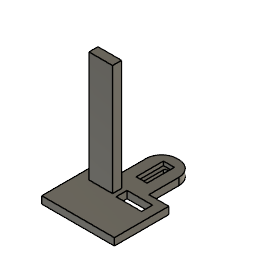
gripperForLego (Autodesk Fusion 360 design; units mm, degrees)
part number: 2026-06-01-16-59-25-849
Autodesk Fusion 360 part; units mm, degrees
sketch "スケッチ1" plane through (0, 0, 0) normal (0, 0, 1) x (1, 0, 0)
  line L0 (0, 0) -> (40, 0)
  line L1 (40, 0) -> (40, 30)
  line L2 (40, 30) -> (0, 30)
  line L3 (0, 30) -> (0, 0)
  line L4 (6, 21) -> (18, 21)
  line L5 (18, 21) -> (18, 25)
  line L6 (18, 25) -> (6, 25)
  line L7 (6, 25) -> (6, 21)
  line L8 (21, 20) -> (35, 20)
  line L9 (35, 20) -> (35, 26)
  line L10 (35, 26) -> (21, 26)
  line L11 (21, 26) -> (21, 20)
  dimension "d1" = 30
  constraint horizontal L0
  constraint vertical L1
  constraint horizontal L2
  constraint vertical L3
  constraint coincident L0.start L3.end
  constraint horizontal L4
  constraint vertical L5
  constraint horizontal L6
  constraint vertical L7
  constraint horizontal L8
  constraint vertical L9
  constraint horizontal L10
  constraint vertical L11
  measures "d1" distance of L0.end L1.end
extrude "押し出し1" add sketch "スケッチ1" along normal blind 4
sketch "スケッチ2" plane through (0, 0, 4) normal (0, 0, 1) x (-1, 0, 0)
  line L0 (-6, -21) -> (-6, -25)
  line L1 (-6, -25) -> (-18, -25)
  line L2 (-18, -25) -> (-18, -21)
  line L3 (-18, -21) -> (-6, -21)
  line L4 (-21, -20) -> (-21, -26)
  line L5 (-21, -26) -> (-35, -26)
  line L6 (-35, -26) -> (-35, -20)
  line L7 (-35, -20) -> (-21, -20)
  line L8 (0, -30) -> (0, 0)
  line L9 (0, 0) -> (-40, 0)
  line L10 (-40, 0) -> (-40, -30)
  line L11 (-40, -30) -> (0, -30)
sketch "スケッチ3" plane through (0, 0, 0) normal (0, 0, -1) x (1, 0, 0)
  line L0 (6, -25) -> (6, -21)
  line L1 (6, -21) -> (18, -21)
  line L2 (18, -21) -> (18, -25)
  line L3 (18, -25) -> (6, -25)
  line L4 (21, -26) -> (21, -20)
  line L5 (21, -20) -> (35, -20)
  line L6 (35, -20) -> (35, -26)
  line L7 (35, -26) -> (21, -26)
  line L8 (0, 0) -> (0, -30)
  line L9 (0, -30) -> (40, -30)
  line L10 (40, -30) -> (40, 0)
  line L11 (40, 0) -> (0, 0)
  line L12 (19, -21) -> (5, -21)
  line L13 (5, -21) -> (5, -26)
  line L14 (5, -26) -> (19, -26)
  line L15 (19, -26) -> (19, -21)
  constraint horizontal L12
  constraint vertical L13
  constraint horizontal L14
  constraint vertical L15
extrude "押し出し2" cut sketch "スケッチ3" against normal blind 1 contours L0 L2 L3 L12 L13 L14 L15
sketch "スケッチ4" plane through (0, 0, 0) normal (0, 0, -1) x (1, 0, 0)
  line L0 (0, 0) -> (0, -30)
  line L1 (0, -30) -> (40, -30)
  line L2 (40, -30) -> (40, 0)
  line L3 (40, 0) -> (0, 0)
  line L4 (21, -26) -> (21, -20)
  line L5 (21, -20) -> (35, -20)
  line L6 (35, -20) -> (35, -26)
  line L7 (35, -26) -> (21, -26)
  line L8 (5, -21) -> (19, -21)
  line L9 (19, -21) -> (19, -26)
  line L10 (19, -26) -> (5, -26)
  line L11 (5, -26) -> (5, -21)
sketch "スケッチ5" plane through (0, 0, 0) normal (0, 0, -1) x (1, 0, 0)
  line L0 (11, -30) -> (29, -30)
  line L1 (29, -30) -> (29, -55)
  line L2 (29, -55) -> (11, -55)
  line L3 (11, -55) -> (11, -30)
  line L4 (19, -48) -> (19, -37)
  line L5 (21, -48) -> (21, -37)
  circle A0 centre (20, -48) radius 1
  circle A1 centre (20, -37) radius 1
  constraint horizontal L0
  constraint vertical L1
  constraint horizontal L2
  constraint vertical L3
  constraint parallel L3 L4
  constraint vertical L5
  constraint coincident L5.start A0
  constraint tangent L5 A0
  constraint coincident L5.end A1
  constraint tangent L5 A1
extrude "押し出し3" add sketch "スケッチ5" against normal blind 4
fillet "フィレット1" radius 8.5 2 edges at (11, 55, 2) (29, 55, 2)
sketch "スケッチ6" plane through (0, 0, 4) normal (0, 0, 1) x (-1, 0, 0)
  line L0 (-19, -21) -> (-5, -21)
  line L1 (-5, -21) -> (-5, -26)
  line L2 (-5, -26) -> (-19, -26)
  line L3 (-19, -26) -> (-19, -21)
  constraint horizontal L0
  constraint vertical L1
  constraint horizontal L2
  constraint vertical L3
extrude "押し出し4" cut sketch "スケッチ6" against normal blind 2
extrude "押し出し5" add sketch "スケッチ4" against normal blind 1 contours L8 L9 L10 L11
extrude "押し出し6" cut sketch "スケッチ2" against normal blind 200 contours L0 L1 L2 L3
sketch "スケッチ7" plane through (0, 0, 4) normal (0, 0, 1) x (-1, 0, 0)
  line L0 (-19, -21) -> (-5, -21)
  line L1 (-5, -21) -> (-5, -26)
  line L2 (-5, -26) -> (-19, -26)
  line L3 (-19, -26) -> (-19, -21)
  arc A0 (-29, -46.5) -> (-20.5, -55) centre (-20.5, -46.5) ccw
  line L4 (-20.5, -55) -> (-19.5, -55)
  arc A1 (-19.5, -55) -> (-11, -46.5) centre (-19.5, -46.5) ccw
  line L5 (-11, -46.5) -> (-11, -30)
  line L6 (-11, -30) -> (0, -30)
  line L7 (0, -30) -> (0, 0)
  line L8 (0, 0) -> (-40, 0)
  line L9 (-40, 0) -> (-40, -30)
  line L10 (-40, -30) -> (-29, -30)
  line L11 (-29, -30) -> (-29, -46.5)
  arc A2 (-21, -48) -> (-19, -48) centre (-20, -48) ccw
  line L12 (-21, -48) -> (-21, -37)
  arc A3 (-19, -37) -> (-21, -37) centre (-20, -37) ccw
  line L13 (-19, -37) -> (-19, -48)
  line L14 (-21, -20) -> (-21, -26)
  line L15 (-21, -26) -> (-35, -26)
  line L16 (-35, -26) -> (-35, -20)
  line L17 (-35, -20) -> (-21, -20)
  line L18 (-17, -50) -> (-23, -50)
  line L19 (-23, -50) -> (-23, -35)
  line L20 (-23, -35) -> (-17, -35)
  line L21 (-17, -35) -> (-17, -50)
  constraint horizontal L18
  constraint vertical L19
  constraint horizontal L20
  constraint vertical L21
extrude "押し出し7" cut sketch "スケッチ7" against normal blind 2.2 contours L18 L19 L20 L21
sketch "スケッチ8" plane through (0, 0, 0) normal (0, 0, -1) x (1, 0, 0)
  line L0 (18, -25) -> (6, -25)
  line L1 (6, -25) -> (6, -21)
  line L2 (6, -21) -> (18, -21)
  line L3 (18, -21) -> (18, -25)
  arc A0 (19, -48) -> (21, -48) centre (20, -48) ccw
  line L4 (19, -48) -> (19, -37)
  arc A1 (21, -37) -> (19, -37) centre (20, -37) ccw
  line L5 (21, -37) -> (21, -48)
  arc A2 (20.5, -55) -> (29, -46.5) centre (20.5, -46.5) ccw
  line L6 (29, -46.5) -> (29, -30)
  line L7 (29, -30) -> (40, -30)
  line L8 (40, -30) -> (40, 0)
  line L9 (40, 0) -> (0, 0)
  line L10 (0, 0) -> (0, -30)
  line L11 (0, -30) -> (11, -30)
  line L12 (11, -30) -> (11, -46.5)
  arc A3 (11, -46.5) -> (19.5, -55) centre (19.5, -46.5) ccw
  line L13 (19.5, -55) -> (20.5, -55)
  line L14 (21, -26) -> (21, -20)
  line L15 (21, -20) -> (35, -20)
  line L16 (35, -20) -> (35, -26)
  line L17 (35, -26) -> (21, -26)
  line L18 (18.5, -25.5) -> (5.5, -25.5)
  line L19 (5.5, -25.5) -> (5.5, -20.5)
  line L20 (5.5, -20.5) -> (18.5, -20.5)
  line L21 (18.5, -20.5) -> (18.5, -25.5)
  line L22 (5, -26) -> (19, -26)
  line L23 (19, -26) -> (19, -21)
  line L24 (19, -21) -> (5, -21)
  line L25 (5, -21) -> (5, -26)
  constraint horizontal L18
  constraint vertical L19
  constraint horizontal L20
  constraint vertical L21
  constraint horizontal L22
  constraint vertical L23
  constraint horizontal L24
  constraint vertical L25
extrude "押し出し8" add 1 faces at (10, 25.6667, 2) along direction (0, 0, 1) blind 2
extrude "押し出し9" add sketch "スケッチ8" against normal blind 65 contours L0 L1 L3 L18 L19 L21 L24 | L0 L1 L2 L3 L24 | L2 L19 L20 L21 L24
